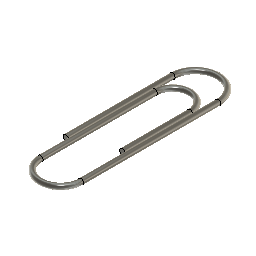
Mech Week 1 v8 (Autodesk Fusion 360 design; units mm, degrees)
Autodesk Fusion 360 part; units mm, degrees
sketch "Sketch10" plane through (0, 0, 0) normal (0, 0, 1) x (1, 0, 0)
  line L0 (50.017, 82.2927) -> (85.017, 21.6709)
  line L1 (85.017, 21.6709) -> (120.017, 82.2927)
  arc A0 (120.017, 82.2927) -> (88.8401, 100.2927) centre (104.4286, 91.2927) ccw
  line L2 (88.8401, 100.2927) -> (85.017, 93.6709)
  line L3 (85.017, 93.6709) -> (81.1939, 100.2927)
  arc A1 (81.1939, 100.2927) -> (50.017, 82.2927) centre (65.6055, 91.2927) ccw
  arc A2 (-6.3191, 110.6896) -> (29.9359, 39.8389) centre (15.4176, 77.1111) ccw
  arc A3 (-6.3191, 110.6896) -> (29.9359, 39.8389) centre (-6.8955, 65.6933) ccw
  circle A4 centre (196.6362, 61.204) radius 45
  line L4 (196.6362, 61.204) -> (227.183, 94.2479)
  line L5 (196.6362, 61.204) -> (229.6801, 30.6573)
  dimension "d34" = 70
  dimension "d35" = 60
  dimension "d36" = 18
  dimension "d37" = 40
  dimension "d38" = 45
  dimension "d40" = 90
  dimension "d41" = 90
  constraint tangent L1 A0
  constraint tangent A0 L2
  constraint parallel L1 L2
  constraint tangent L3 A1
  constraint equal A0 A1
  constraint equal L2 L3
  constraint equal L0 L1
  constraint tangent L0 A1
  constraint vertical L0.end L2.end
  constraint coincident A4.centre L4.start
  constraint coincident A4 L4.end
  constraint coincident A4 L5.end
  measures "d34" distance of L0.end L1.end
  measures "d35" angle of L0 L1
  measures "d36" radius of A1
  measures "d37" radius of A2
  measures "d38" radius of A3
  measures "d40" diameter of A4
  measures "d41" angle of L4 L5
extrude "Extrude6" add sketch "Sketch10" along normal blind 20 contours L0 L1 A0 L2 L3 A1 | A2 A3 | A4 L4 L5 picked at (176.8722, 38.7426) makes body 1 at (176.8722, 38.7426, 0) makes body 2 at (73.3504, 65.8782, 0) makes body 3 at (-24.9278, 24.4642, 13.3333)
sketch "Sketch1" plane through (0, 0, 0) normal (0, 0, 1) x (1, 0, 0)
  line L0 (0, 0) -> (60, 0)
  line L1 (60, 0) -> (60, 60)
  line L2 (60, 60) -> (0, 60)
  line L3 (0, 60) -> (0, 0)
  dimension "d8" = 60
  dimension "d9" = 60
  constraint horizontal L0
  constraint vertical L1
  constraint horizontal L2
  constraint vertical L3
  constraint coincident L0.start L3.end
  measures "d8" distance of L0.start L0.end
  measures "d9" distance of L0.start L2.end
extrude "Extrude1" add sketch "Sketch1" along normal blind 60 separate body makes body 4
sketch "Sketch2" plane through (0, 0, 0) normal (0, -1, 0) x (1, 0, 0)
  line L0 (0, 0) -> (60, 0)
  line L1 (60, 0) -> (60, 60)
  line L2 (60, 60) -> (0, 60)
  line L3 (0, 60) -> (0, 0)
  line L4 (60, 60) -> (0, 0) construction
  circle A0 centre (30, 30) radius 15
  dimension "d12" = 30
  constraint coincident L1.end L2.start
  constraint coincident L0.start L3.end
  constraint midpoint L4 A0.centre
  measures "d12" diameter of A0
extrude "Extrude2" cut sketch "Sketch2" against normal blind 7 contours A0 bodies 4
sketch "Sketch3" plane through (60, 0, 0) normal (1, 0, 0) x (0, 1, 0)
  line L0 (0, 0) -> (60, 0)
  line L1 (60, 0) -> (60, 60)
  line L2 (60, 60) -> (0, 60)
  line L3 (0, 60) -> (0, 0)
  line L4 (60, 60) -> (0, 0) construction
  line L5 (45, 38.6603) -> (30, 47.3205)
  line L6 (30, 47.3205) -> (15, 38.6603)
  line L7 (15, 38.6603) -> (15, 21.3397)
  line L8 (15, 21.3397) -> (30, 12.6795)
  line L9 (30, 12.6795) -> (45, 21.3397)
  line L10 (45, 21.3397) -> (45, 38.6603)
  point P0 (30, 30)
  dimension "d15" = 15
  constraint coincident L1.end L2.start
  constraint coincident L0.start L3.end
  constraint midpoint L4 P0
  constraint vertical L10
  measures "d15" distance of P0 L10
extrude "Extrude3" cut sketch "Sketch3" against normal blind 10 contours L5 L6 L7 L8 L9 L10 bodies 4
sketch "Sketch4" plane through (0, 0, 60) normal (0, 0, 1) x (-1, 0, 0)
  line L0 (0, -60) -> (0, 0)
  line L1 (0, 0) -> (-60, 0)
  line L2 (-60, 0) -> (-60, -60)
  line L3 (-60, -60) -> (0, -60)
  line L4 (-15, -45) -> (-15, -15)
  line L5 (-15, -15) -> (-45, -15)
  line L6 (-45, -15) -> (-45, -45)
  line L7 (-45, -45) -> (-15, -45)
  dimension "d18" = -15
extrude "Extrude4" cut sketch "Sketch4" against normal blind 8 contours L4 L5 L6 L7 bodies 4
sketch "Activity3" plane through (0, 0, 0) normal (0, 0, 1) x (1, 0, 0)
  line L0 (0, 0) -> (30.9017, 95.1057)
  line L1 (30.9017, 95.1057) -> (61.8034, 0)
  line L2 (61.8034, 0) -> (-19.0983, 58.7785)
  line L3 (-19.0983, 58.7785) -> (80.9017, 58.7785)
  line L4 (80.9017, 58.7785) -> (0, 0)
  dimension "d21" = 36
  dimension "d23" = 100
  constraint coincident L0.start L4.end
  constraint horizontal L3
  constraint equal L0 L2
  constraint equal L0 L1
  constraint equal L1 L4
  constraint equal L3 L4
  constraint horizontal L0.start L1.end
  measures "d21" angle of L0 L4
  measures "d23" distance of L2.end L3.end
sketch "Sketch7" plane through (0, 0, 0) normal (0, 0, 1) x (1, 0, 0)
  line L0 (0, 0) -> (100, 0)
  line L1 (100, 0) -> (100, 100)
  line L2 (100, 100) -> (0, 100)
  line L3 (0, 100) -> (0, 0)
  dimension "d24" = 100
  dimension "d25" = 100
  constraint horizontal L0
  constraint vertical L1
  constraint horizontal L2
  constraint vertical L3
  constraint coincident L0.start L3.end
  measures "d24" distance of L0.start L0.end
  measures "d25" distance of L0.start L2.end
extrude "Extrude5" add sketch "Sketch7" along normal blind 50 draft -45 separate body makes body 5
sketch "Sketch9" plane through (0, 0, 0) normal (0, 1, 0) x (1, 0, 0)
  line L0 (0, -51.9615) -> (0, 0)
  line L1 (0, 0) -> (30, 0)
  line L2 (30, 0) -> (0, -51.9615)
  dimension "d31" = 60
  dimension "d32" = 30
  constraint coincident L0.end L1.start
  constraint vertical L0
  constraint perpendicular L0 L1
  measures "d31" angle of L1 L2
  measures "d32" distance of L0.end L1.end
revolve "Revolve1" add sketch "Sketch9" angle 360 about axis through (0, 0, 51.9615) along (0, 0, -1) separate body makes body 6
sketch "Sketch15" plane through (0, 0, 0) normal (0, 0, 1) x (1, 0, 0)
  line L0 (0, 0) -> (0, 140)
  arc A0 (60, 140) -> (0, 140) centre (30, 140) ccw
  line L1 (60, 140) -> (60, -40)
  arc A1 (7, -40) -> (60, -40) centre (33.5, -40) ccw
  line L2 (7, -40) -> (7, 110)
  arc A2 (53, 110) -> (7, 110) centre (30, 110) ccw
  line L3 (53, 110) -> (53, 21.1942)
  dimension "d68" = 7
  dimension "d69" = 7
  dimension "d71" = 30
  dimension "d72" = 30
  dimension "d73" = 180
  dimension "d74" = 40
  constraint coincident L0.start origin
  constraint vertical L0
  constraint tangent L0 A0
  constraint tangent A0 L1
  constraint parallel L0 L1
  constraint tangent L1 A1
  constraint tangent A1 L2
  constraint parallel L1 L2
  constraint tangent L2 A2
  constraint tangent A2 L3
  constraint parallel L2 L3
  measures "d68" distance of L0 L2
  measures "d69" distance of L1 L3
  measures "d9" radius of A0
  measures "d72" distance of A0.centre A2.centre
  measures "d73" vertical distance of A0.centre A1.centre
  measures "d74" vertical distance of L0.start A1.centre
ref_plane "WorkPlane2" through (0, 0, 0) normal (0, 1, 0) x (-1, 0, 0)
sketch "Sketch16" plane through (0, 0, 0) normal (0, 1, 0) x (-1, 0, 0)
  circle A0 centre (0, 0) radius 3.5
  dimension "d76" = 7
  constraint coincident A0.centre origin
  measures "d76" diameter of A0
sweep "Sweep2" add profiles "Sketch16" path "Sketch15" along L0 A0 L1 A1 L2 A2 L3 section 1 separate body makes body 7
hidden bodies 1 2 3 4 5 6
named bodies: "Activity2", "Activity4.2", "Activity4.1", "Activity1", "Activity1 (1)", "Activity1 (2)", "Activity5"
